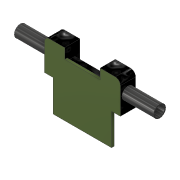
# Autodesk Inventor part: flowMeter
Saved by Autodesk Inventor 2019 (Build 230136000, 136)
## iProperties
Created: 2020-10-21
Part Number: flowMeter
Material: Generic
Document SubType Name: Modeling
Designer: UCLA
Density: 1 g/cm^3
Appearance: Black
Author: UCLA
Autodesk Inventor part; units mm, degrees
ref_plane "YZ Plane" through (0, 0, 0) normal (1, 0, 0) x (0, 1, 0)
ref_plane "XZ Plane" through (0, 0, 0) normal (0, 1, 0) x (-1, 0, 0)
ref_plane "XY Plane" through (0, 0, 0) normal (0, 0, 1) x (1, 0, 0)
sketch "Sketch2" plane through (0, 0, 0) normal (0, 0, 1) x (1, 0, 0)
  line L0 (11.5, -10.5) -> (-11.5, -10.5)
  line L1 (-11.5, -10.5) -> (-11.5, 10.5)
  line L2 (-11.5, 10.5) -> (11.5, 10.5)
  line L3 (11.5, 10.5) -> (11.5, -10.5)
  line L4 (11.5, -10.5) -> (-11.5, 10.5) construction
  line L5 (-11.5, -10.5) -> (11.5, 10.5) construction
  point P0 (0, 0)
  dimension "d0" = 23
  dimension "d1" = 21
  constraints: 12 end point, 2 midpoint, 2 parallel, 1 horizontal, 1 perpendicular
  measures "d0" distance of L1.end L2.end
  measures "d1" distance of L0.end L1.end
extrude "Extrusion1" add sketch "Sketch2" along normal blind 1
sketch "Sketch3" plane through (0, 0, 1) normal (0, 0, 1) x (1, 0, 0)
  line L0 (-7, 14.5) -> (-13, 14.5)
  line L1 (-15, 12.5) -> (-15, 2)
  line L2 (-15, 2) -> (-7, 2)
  line L3 (-7, 2) -> (-7, 14.5)
  line L4 (7, 14.5) -> (13, 14.5)
  line L5 (15, 12.5) -> (15, 2)
  line L6 (15, 2) -> (7, 2)
  line L7 (7, 2) -> (7, 14.5)
  line L8 (-7, 14.5) -> (7, 14.5) construction
  line L9 (0, 14.5) -> (0, 0) construction
  arc A0 (-13, 14.5) -> (-15, 12.5) centre (-13, 12.5) ccw
  arc A1 (15, 12.5) -> (13, 14.5) centre (13, 12.5) ccw
  line L10 (11.5, -10.5) -> (-11.5, -10.5) projected
  dimension "d5" = 14
  dimension "d6" = 8
  dimension "d7" = 8
  dimension "d9" = 12.5
  dimension "d10" = 2
  dimension "d20" = 12.5
  constraints: 20 end point, 4 parallel, 4 point on circle, 4 tangent, 2 centre point, 2 horizontal, 2 perpendicular, 2 point on line, 1 equal radius, 1 midpoint, 1 vertical
  measures "d5" distance between parallel lines of L7 L3
  measures "d6" distance between parallel lines of L3 L1
  measures "d7" distance between parallel lines of L7 L5
  measures "d9" distance between parallel lines of L4 L6
  measures "d10" radius of A0
  measures "d20" distance between parallel lines of L10 L6
extrude "Extrusion2" add sketch "Sketch3" against normal blind 6
sketch "Sketch6" plane through (0, 0, 0) normal (0, 0, -1) x (-1, 0, 0)
  line L0 (-7, 9.5) -> (7, 9.5)
  line L1 (7, 9.5) -> (7, 2)
  line L2 (7, 2) -> (-7, 2)
  line L3 (-7, 2) -> (-7, 9.5)
  line L4 (-5, 2) -> (5, 2)
  line L5 (5, 2) -> (5, -2)
  line L6 (5, -2) -> (-5, -2)
  line L7 (-5, -2) -> (-5, 2)
  line L8 (-7, 10.5) -> (-7, 2) projected
  line L9 (7, 10.5) -> (-7, 10.5) projected
  point P0 (0, 0)
  dimension "d23" = 4
  dimension "d27" = 2
  dimension "d28" = 1
  dimension "d29" = 2
  constraints: 17 end point, 4 parallel, 3 perpendicular, 2 horizontal, 1 collinear, 1 point on line
  measures "d23" distance between parallel lines of L2 L6
  measures "d27" distance between parallel lines of L3 L7
  measures "d28" distance between parallel lines of L9 L0
  measures "d29" distance between parallel lines of L1 L5
extrude "Extrusion5" add sketch "Sketch6" along normal blind 3
sketch "Sketch4" plane through (15, 2, 1) normal (1, 0, 0) x (0, 0, -1)
  line L0 (0, 10.5) -> (6, 10.5) projected
  line L1 (3, 10.5) -> (3, 2.5) construction
  circle A0 centre (3, 6.5) radius 2.4
  circle A1 centre (3, 6.5) radius 2
  point P0 (1, -2)
  point P1 (0, 8)
  dimension "d13" = 4.8
  dimension "d14" = 4
  dimension "d15" = 4
  constraints: 2 centre point, 2 end point, 1 coincident, 1 midpoint, 1 vertical, 2 other
  measures "d13" diameter of A0
  measures "d14" diameter of A1
extrude "Extrusion3" add sketch "Sketch4" along normal blind 12.5
sketch "Sketch5" plane through (-15, 2, 1) normal (-1, 0, 0) x (0, 0, 1)
  circle A0 centre (-3, 6.5) radius 2.4 projected
  circle A1 centre (-3, 6.5) radius 2 projected
  point P0 (-1, -2)
extrude "Extrusion4" add sketch "Sketch5" along normal blind 12.5
body "Solid1"
